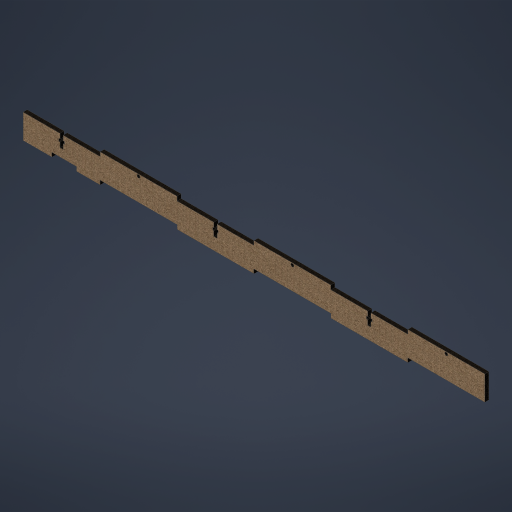
# Autodesk Inventor part: Cableduct_Side
Saved by Autodesk Inventor 2024.1 (Build 281209000, 209)
## iProperties
Created: 2023-08-04
Part Number: Cableduct_Side
Material: MDF Medium Density Fiberboard
Document SubType Name: Modeling
Designer: jaege
Density: 0.8 g/cm^3
Appearance: Cardboard - Corrugated
Author: jaege
Autodesk Inventor part; units mm, degrees
ref_plane "YZ Plane" through (0, 0, 0) normal (1, 0, 0) x (0, 1, 0)
ref_plane "XZ Plane" through (0, 0, 0) normal (0, 1, 0) x (-1, 0, 0)
ref_plane "XY Plane" through (0, 0, 0) normal (0, 0, 1) x (1, 0, 0)
sketch "Sketch1" plane through (0, 0, 0) normal (0, 0, 1) x (1, 0, 0)
  line L0 (-300, -24) -> (-300, -20) projected
  line L1 (-225, -24) -> (-300, -24) construction
  line L2 (-225, -20) -> (-225, -24) projected
  line L3 (-225, -20) -> (-300, -20) projected
  line L4 (-150, -24) -> (-150, -20) projected
  line L5 (-75, -24) -> (-150, -24) construction
  line L6 (-75, -20) -> (-75, -24) projected
  line L7 (-75, -20) -> (-150, -20) projected
  circle A0 centre (-262.5, 2) radius 1.5 projected
  circle A1 centre (-112.5, 2) radius 1.5 projected
  circle A2 centre (37.5, 2) radius 1.5 projected
  line L8 (-236, -49) -> (-236, -199) construction
  line L9 (-236, -199) -> (11, -199) construction
  line L10 (11, -199) -> (11, -49) construction
  line L11 (11, -49) -> (-236, -49) construction
  circle A3 centre (43, -151.5) radius 1.5 construction
  circle A4 centre (43, -96.5) radius 1.5 construction
  circle A5 centre (-268, -96.5) radius 1.5 construction
  circle A6 centre (-268, -151.5) radius 1.5 construction
  circle A7 centre (-335, -151.5) radius 1.5 construction
  circle A8 centre (-335, -96.5) radius 1.5 construction
  line L12 (-270, -161.5) -> (-270, -196.5) construction
  line L13 (-270, -196.5) -> (-266, -196.5) construction
  line L14 (-266, -196.5) -> (-266, -161.5) construction
  line L15 (-266, -161.5) -> (-270, -161.5) construction
  line L16 (45, -51.5) -> (41, -51.5) construction
  line L17 (41, -51.5) -> (41, -86.5) construction
  line L18 (41, -86.5) -> (45, -86.5) construction
  line L19 (45, -86.5) -> (45, -51.5) construction
  line L20 (45, -141.5) -> (45, -106.5) construction
  line L21 (45, -106.5) -> (41, -106.5) construction
  line L22 (41, -106.5) -> (41, -141.5) construction
  line L23 (41, -141.5) -> (45, -141.5) construction
  line L24 (-337, -161.5) -> (-337, -196.5) construction
  line L25 (-337, -196.5) -> (-333, -196.5) construction
  line L26 (-333, -196.5) -> (-333, -161.5) construction
  line L27 (-333, -161.5) -> (-337, -161.5) construction
  line L28 (-270, -106.5) -> (-270, -141.5) construction
  line L29 (-270, -141.5) -> (-266, -141.5) construction
  line L30 (-266, -141.5) -> (-266, -106.5) construction
  line L31 (-266, -106.5) -> (-270, -106.5) construction
  line L32 (-337, -51.5) -> (-337, -86.5) construction
  line L33 (-337, -86.5) -> (-333, -86.5) construction
  line L34 (-333, -86.5) -> (-333, -51.5) construction
  line L35 (-333, -51.5) -> (-337, -51.5) construction
  line L36 (41, -161.5) -> (41, -196.5) construction
  line L37 (41, -196.5) -> (45, -196.5) construction
  line L38 (45, -196.5) -> (45, -161.5) construction
  line L39 (45, -161.5) -> (41, -161.5) construction
  line L40 (-333, -106.5) -> (-337, -106.5) construction
  line L41 (-337, -106.5) -> (-337, -141.5) construction
  line L42 (-337, -141.5) -> (-333, -141.5) construction
  line L43 (-333, -141.5) -> (-333, -106.5) construction
  line L44 (-266, -51.5) -> (-270, -51.5) construction
  line L45 (-270, -51.5) -> (-270, -86.5) construction
  line L46 (-270, -86.5) -> (-266, -86.5) construction
  line L47 (-266, -86.5) -> (-266, -51.5) construction
  circle A9 centre (-112.5, -226) radius 1.5 construction
  circle A10 centre (-262.5, -226) radius 1.5 construction
  circle A11 centre (-187.5, -22) radius 1.5 construction
  circle A12 centre (-37.5, -22) radius 1.5 construction
  circle A13 centre (-337.5, -22) radius 1.5 construction
  circle A14 centre (37.5, -226) radius 1.5 construction
  line L48 (-375, -36.5) -> (-375, 0) projected
  line L49 (-336, 0) -> (-300, 0) projected
  line L50 (-300, 0) -> (-300, 4) projected
  line L51 (-300, 4) -> (-225, 4) projected
  line L52 (-225, 4) -> (-225, 0) projected
  line L53 (-225, 0) -> (-189, 0) projected
  line L54 (-150, 0) -> (-150, 4) projected
  line L55 (-150, 4) -> (-75, 4) projected
  line L56 (-75, 4) -> (-75, 0) projected
  line L57 (-75, 0) -> (-39, 0) projected
  line L58 (0, 0) -> (0, 4) projected
  line L59 (0, 4) -> (75, 4) projected
  line L60 (75, 4) -> (75, -20) projected
  line L61 (75, -20) -> (0, -20) projected
  line L62 (0, -24) -> (0, -20) projected
  line L63 (75, -24) -> (0, -24) construction
  line L64 (75, -36.5) -> (75, -24) projected
  line L65 (79, -36.5) -> (75, -36.5) projected
  line L66 (79, -71.5) -> (79, -36.5) construction
  line L67 (75, -71.5) -> (79, -71.5) construction
  line L68 (75, -87.5) -> (75, -71.5) construction
  line L69 (70.2, -87.5) -> (75, -87.5) construction
  line L70 (70.2, -86.3) -> (70.2, -87.5) construction
  line L71 (67.8, -86.3) -> (70.2, -86.3) construction
  line L72 (67.8, -87.5) -> (67.8, -86.3) construction
  line L73 (63, -87.5) -> (67.8, -87.5) construction
  line L74 (63, -90.5) -> (63, -87.5) construction
  line L75 (67.8, -90.5) -> (63, -90.5) construction
  line L76 (67.8, -91.7) -> (67.8, -90.5) construction
  line L77 (70.2, -91.7) -> (67.8, -91.7) construction
  line L78 (70.2, -90.5) -> (70.2, -91.7) construction
  line L79 (75, -90.5) -> (70.2, -90.5) construction
  line L80 (75, -106.5) -> (75, -90.5) construction
  line L81 (79, -106.5) -> (75, -106.5) construction
  line L82 (79, -141.5) -> (79, -106.5) construction
  line L83 (75, -141.5) -> (79, -141.5) construction
  line L84 (75, -157.5) -> (75, -141.5) construction
  line L85 (70.2, -157.5) -> (75, -157.5) construction
  line L86 (70.2, -156.3) -> (70.2, -157.5) construction
  line L87 (67.8, -156.3) -> (70.2, -156.3) construction
  line L88 (67.8, -157.5) -> (67.8, -156.3) construction
  line L89 (63, -157.5) -> (67.8, -157.5) construction
  line L90 (63, -160.5) -> (63, -157.5) construction
  line L91 (67.8, -160.5) -> (63, -160.5) construction
  line L92 (67.8, -161.7) -> (67.8, -160.5) construction
  line L93 (70.2, -161.7) -> (67.8, -161.7) construction
  line L94 (70.2, -160.5) -> (70.2, -161.7) construction
  line L95 (75, -160.5) -> (70.2, -160.5) construction
  line L96 (75, -176.5) -> (75, -160.5) construction
  line L97 (79, -176.5) -> (75, -176.5) construction
  line L98 (79, -211.5) -> (79, -176.5) construction
  line L99 (75, -211.5) -> (79, -211.5) construction
  line L100 (75, -228) -> (75, -211.5) construction
  line L101 (0, -228) -> (75, -228) construction
  line L102 (0, -224) -> (0, -228) construction
  line L103 (-36, -224) -> (0, -224) construction
  line L104 (-36, -224) -> (-36, -219.2) construction
  line L105 (-36, -219.2) -> (-34.8, -219.2) construction
  line L106 (-34.8, -219.2) -> (-34.8, -216.8) construction
  line L107 (-34.8, -216.8) -> (-36, -216.8) construction
  line L108 (-36, -216.8) -> (-36, -212) construction
  line L109 (-36, -212) -> (-39, -212) construction
  line L110 (-39, -212) -> (-39, -216.8) construction
  line L111 (-39, -216.8) -> (-40.2, -216.8) construction
  line L112 (-40.2, -216.8) -> (-40.2, -219.2) construction
  line L113 (-40.2, -219.2) -> (-39, -219.2) construction
  line L114 (-39, -219.2) -> (-39, -224) construction
  line L115 (-75, -224) -> (-39, -224) construction
  line L116 (-75, -228) -> (-75, -224) construction
  line L117 (-150, -228) -> (-75, -228) construction
  line L118 (-150, -224) -> (-150, -228) construction
  line L119 (-186, -224) -> (-150, -224) construction
  line L120 (-186, -224) -> (-186, -219.2) construction
  line L121 (-186, -219.2) -> (-184.8, -219.2) construction
  line L122 (-184.8, -219.2) -> (-184.8, -216.8) construction
  line L123 (-184.8, -216.8) -> (-186, -216.8) construction
  line L124 (-186, -216.8) -> (-186, -212) construction
  line L125 (-186, -212) -> (-189, -212) construction
  line L126 (-189, -212) -> (-189, -216.8) construction
  line L127 (-189, -216.8) -> (-190.2, -216.8) construction
  line L128 (-190.2, -216.8) -> (-190.2, -219.2) construction
  line L129 (-190.2, -219.2) -> (-189, -219.2) construction
  line L130 (-189, -219.2) -> (-189, -224) construction
  line L131 (-225, -224) -> (-189, -224) construction
  line L132 (-225, -228) -> (-225, -224) construction
  line L133 (-300, -228) -> (-225, -228) construction
  line L134 (-300, -224) -> (-300, -228) construction
  line L135 (-336, -224) -> (-300, -224) construction
  line L136 (-336, -224) -> (-336, -219.2) construction
  line L137 (-336, -219.2) -> (-334.8, -219.2) construction
  line L138 (-334.8, -219.2) -> (-334.8, -216.8) construction
  line L139 (-334.8, -216.8) -> (-336, -216.8) construction
  line L140 (-336, -216.8) -> (-336, -212) construction
  line L141 (-336, -212) -> (-339, -212) construction
  line L142 (-339, -212) -> (-339, -216.8) construction
  line L143 (-339, -216.8) -> (-340.2, -216.8) construction
  line L144 (-340.2, -216.8) -> (-340.2, -219.2) construction
  line L145 (-340.2, -219.2) -> (-339, -219.2) construction
  line L146 (-339, -219.2) -> (-339, -224) construction
  line L147 (-375, -224) -> (-339, -224) construction
  line L148 (-375, -211.5) -> (-375, -224) construction
  line L149 (-383, -211.5) -> (-375, -211.5) construction
  line L150 (-383, -176.5) -> (-383, -211.5) construction
  line L151 (-375, -176.5) -> (-383, -176.5) construction
  line L152 (-375, -160.5) -> (-375, -176.5) construction
  line L153 (-370.2, -160.5) -> (-375, -160.5) construction
  line L154 (-370.2, -161.7) -> (-370.2, -160.5) construction
  line L155 (-367.8, -161.7) -> (-370.2, -161.7) construction
  line L156 (-367.8, -160.5) -> (-367.8, -161.7) construction
  line L157 (-363, -160.5) -> (-367.8, -160.5) construction
  line L158 (-363, -157.5) -> (-363, -160.5) construction
  line L159 (-367.8, -157.5) -> (-363, -157.5) construction
  line L160 (-367.8, -156.3) -> (-367.8, -157.5) construction
  line L161 (-370.2, -156.3) -> (-367.8, -156.3) construction
  line L162 (-370.2, -157.5) -> (-370.2, -156.3) construction
  line L163 (-375, -157.5) -> (-370.2, -157.5) construction
  line L164 (-375, -141.5) -> (-375, -157.5) construction
  line L165 (-383, -141.5) -> (-375, -141.5) construction
  line L166 (-383, -106.5) -> (-383, -141.5) construction
  line L167 (-375, -106.5) -> (-383, -106.5) construction
  line L168 (-375, -90.5) -> (-375, -106.5) construction
  line L169 (-370.2, -90.5) -> (-375, -90.5) construction
  line L170 (-370.2, -91.7) -> (-370.2, -90.5) construction
  line L171 (-367.8, -91.7) -> (-370.2, -91.7) construction
  line L172 (-367.8, -90.5) -> (-367.8, -91.7) construction
  line L173 (-363, -90.5) -> (-367.8, -90.5) construction
  line L174 (-363, -87.5) -> (-363, -90.5) construction
  line L175 (-367.8, -87.5) -> (-363, -87.5) construction
  line L176 (-367.8, -86.3) -> (-367.8, -87.5) construction
  line L177 (-370.2, -86.3) -> (-367.8, -86.3) construction
  line L178 (-370.2, -87.5) -> (-370.2, -86.3) construction
  line L179 (-375, -87.5) -> (-370.2, -87.5) construction
  line L180 (-375, -71.5) -> (-375, -87.5) construction
  line L181 (-383, -71.5) -> (-375, -71.5) construction
  line L182 (-383, -36.5) -> (-383, -71.5) construction
  line L183 (-375, -36.5) -> (-383, -36.5) projected
  line L184 (-300, -24) -> (-323, -24)
  line L185 (-225, -24) -> (-150, -24)
  line L186 (-75, -24) -> (0, -24)
  line L187 (-337, -86.5) -> (-337, -51.5) projected
  line L188 (-337, -51.5) -> (-333, -51.5) projected
  line L189 (-333, -86.5) -> (-333, -51.5) projected
  line L190 (-337, -86.5) -> (-333, -86.5) projected
  line L191 (-333, -51.5) -> (-337, -51.5) projected
  line L192 (-337, -20) -> (-333, -20) projected
  line L193 (-337, -20) -> (-347, -20)
  line L194 (-347, -20) -> (-347, -24)
  line L195 (-333, -20) -> (-323, -20)
  line L196 (-323, -20) -> (-323, -24)
  line L197 (-347, -24) -> (-375, -24)
  line L198 (-323, -24) -> (-347, -24) construction
  line L199 (-336, -4.8) -> (-336, 0) projected
  line L200 (-189, 0) -> (-189, -4.8) projected
  line L201 (-189, -4.8) -> (-190.2, -4.8) projected
  line L202 (-190.2, -4.8) -> (-190.2, -7.2) projected
  line L203 (-190.2, -7.2) -> (-189, -7.2) projected
  line L204 (-189, -7.2) -> (-189, -12) projected
  line L205 (-189, -12) -> (-186, -12) projected
  line L206 (-186, -12) -> (-186, -7.2) projected
  line L207 (-186, -7.2) -> (-184.8, -7.2) projected
  line L208 (-184.8, -7.2) -> (-184.8, -4.8) projected
  line L209 (-184.8, -4.8) -> (-186, -4.8) projected
  line L210 (-186, -4.8) -> (-186, 0) projected
  line L211 (-186, 0) -> (-150, 0) projected
  line L212 (-39, 0) -> (-39, -4.8) projected
  line L213 (-39, -4.8) -> (-40.2, -4.8) projected
  line L214 (-40.2, -4.8) -> (-40.2, -7.2) projected
  line L215 (-40.2, -7.2) -> (-39, -7.2) projected
  line L216 (-39, -7.2) -> (-39, -12) projected
  line L217 (-39, -12) -> (-36, -12) projected
  line L218 (-36, -12) -> (-36, -7.2) projected
  line L219 (-36, -7.2) -> (-34.8, -7.2) projected
  line L220 (-34.8, -7.2) -> (-34.8, -4.8) projected
  line L221 (-34.8, -4.8) -> (-36, -4.8) projected
  line L222 (-36, -4.8) -> (-36, 0) projected
  line L223 (-36, 0) -> (0, 0) projected
  line L224 (-339, 0) -> (-339, -4.8) projected
  line L225 (-339, -4.8) -> (-340.2, -4.8) projected
  line L226 (-340.2, -4.8) -> (-340.2, -7.2) projected
  line L227 (-340.2, -7.2) -> (-339, -7.2) projected
  line L228 (-339, -7.2) -> (-339, -12) projected
  line L229 (-339, -12) -> (-336, -12) projected
  line L230 (-336, -12) -> (-336, -7.2) projected
  line L231 (-336, -7.2) -> (-334.8, -7.2) projected
  line L232 (-334.8, -7.2) -> (-334.8, -4.8) projected
  line L233 (-334.8, -4.8) -> (-336, -4.8) projected
  line L234 (-264, -14.6161) -> (-264, -20)
  line L235 (-261, -20) -> (-261, -14.6161)
  line L236 (-261, -14.6161) -> (-259.8, -14.6161)
  line L237 (-259.8, -14.6161) -> (-259.8, -12.2161)
  line L238 (-259.8, -12.2161) -> (-261, -12.2161)
  line L239 (-261, -12.2161) -> (-261, -8)
  line L240 (-261, -8) -> (-264, -8)
  line L241 (-264, -8) -> (-264, -12.2161)
  line L242 (-264, -12.2161) -> (-265.2, -12.2161)
  line L243 (-265.2, -12.2161) -> (-265.2, -14.6161)
  line L244 (-265.2, -14.6161) -> (-264, -14.6161)
  line L245 (-115.2, -12.2161) -> (-115.2, -14.6161)
  line L246 (-115.2, -14.6161) -> (-114, -14.6161)
  line L247 (-111, -20) -> (-111, -14.6161)
  line L248 (-114, -12.2161) -> (-115.2, -12.2161)
  line L249 (-114, -8) -> (-114, -12.2161)
  line L250 (-111, -14.6161) -> (-109.8, -14.6161)
  line L251 (-109.8, -14.6161) -> (-109.8, -12.2161)
  line L252 (-109.8, -12.2161) -> (-111, -12.2161)
  line L253 (-111, -8) -> (-114, -8)
  line L254 (-111, -12.2161) -> (-111, -8)
  line L255 (-114, -14.6161) -> (-114, -20)
  line L256 (34.8, -12.2161) -> (34.8, -14.6161)
  line L257 (34.8, -14.6161) -> (36, -14.6161)
  line L258 (39, -20) -> (39, -14.6161)
  line L259 (36, -12.2161) -> (34.8, -12.2161)
  line L260 (36, -8) -> (36, -12.2161)
  line L261 (39, -14.6161) -> (40.2, -14.6161)
  line L262 (40.2, -14.6161) -> (40.2, -12.2161)
  line L263 (40.2, -12.2161) -> (39, -12.2161)
  line L264 (39, -8) -> (36, -8)
  line L265 (39, -12.2161) -> (39, -8)
  line L266 (36, -14.6161) -> (36, -20)
  line L267 (-375, 0) -> (-339, 0) projected
  point P0 (-262.5, -8)
  point P1 (-262.5, -20)
  point P2 (-112.5, -20)
  point P3 (-112.5, -8)
  point P4 (37.5, -20)
  point P5 (37.5, -8)
  dimension "d2" = 10
  dimension "d3" = 10
  dimension "d4" = 3
  dimension "d5" = 5.4
  dimension "d6" = 12
  dimension "d7" = 2.4
  dimension "d10" = 150
  constraints: 84 end point, 10 horizontal, 6 perpendicular, 6 vertical, 5 collinear, 4 horizontal alignment, 3 vertical alignment, 2 midpoint, 2 point on line, 50 other
  measures "d2" distance of L192.start L193.end
  measures "d3" distance of L192.end L195.end
  measures "d4" distance of L240.start L241.start
  measures "d5" distance of L238.start L243.start
  measures "d6" distance of L234.end L241.start
  measures "d7" distance of L237.start L238.start
  measures "d10" distance of L243.end L245.end
extrude "Extrusion1" add sketch "Sketch1" along normal blind 4 contours L184 L196 L195 L192 L193 L194 L197 L48 L267 L224 L225 L226 L227 L228 L229 L230 L231 L232 L233 L199 L49 L50 L51 L52 L53 L200 L201 L202 L203 L204 L205 L206 L207 L208 L209 L210 L211 L54 L55 L56 L57 L212 L213 L214 L215 L216 L217 L218 L219 L220 L221 L222 L223 L58 L59 L60 L61 L258 L261 L262 L263 L265 L264 L260 L259 L256 L257 L266 L62 L186 L6 L7 L247 L250 L251 L252 L254 L253 L249 L248 L245 L246 L255 L4 L185 L2 L3 L235 L236 L237 L238 L239 L240 L241 L242 L243 L244 L234 L0 | L234 L244 L243 L242 L241 L240 L239 L238 L237 L236 L235 L3 | L255 L246 L245 L248 L249 L253 L254 L252 L251 L250 L247 L7 | L266 L257 L256 L259 L260 L264 L265 L263 L262 L261 L258 L61
body "Solid1"
